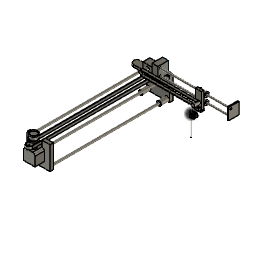
2 D PLOTTER v1 (Autodesk Fusion 360 design; units mm, degrees)
Autodesk Fusion 360 part; units mm, degrees
sketch "Sketch1" plane through (0, 0, 0) normal (0, 1, 0) x (1, 0, 0)
  line L0 (0, 0) -> (100, 0)
  line L1 (100, 0) -> (100, 100)
  line L2 (100, 100) -> (0, 100)
  line L3 (0, 100) -> (0, 0)
  dimension "d1" = 100
  dimension "d2" = 100
  constraint coincident L0.start L3.end
  constraint horizontal L0
  constraint perpendicular L0 L1
  constraint perpendicular L1 L2
  constraint perpendicular L0 L3
  measures "d1" distance of L0.start L0.end
  measures "d2" distance of L0.end L1.end
extrude "Extrude1" add sketch "Sketch1" along normal blind 15 makes body 1
sketch "Sketch2" plane through (0, 0, 0) normal (0, -1, 0) x (1, 0, 0)
  line L0 (0, 0) -> (0, -100)
  line L1 (0, -100) -> (100, -100)
  line L2 (100, -100) -> (100, 0)
  line L3 (100, 0) -> (0, 0)
  line L4 (35, -25) -> (65, -25)
  line L5 (75, -75) -> (75, -35)
  line L6 (25, -35) -> (25, -75)
  line L7 (25, -75) -> (75, -75)
  arc A0 (35, -25) -> (25, -35) centre (35, -35) ccw
  arc A1 (75, -35) -> (65, -25) centre (65, -35) ccw
  dimension "d5" = 10
  constraint parallel L1 L4
  constraint perpendicular L4 L5
  constraint perpendicular L4 L6
  constraint perpendicular L5 L7
  constraint tangent L4 A0
  constraint tangent L6 A0
  constraint tangent L4 A1
  constraint tangent L5 A1
  constraint equal A0 A1
  measures "d5" radius of A0
extrude "Extrude2" add sketch "Sketch2" along normal blind 40 contours L4 L5 L6 L7 A0 A1 bodies 1
sketch "Sketch3" plane through (0, 0, -25) normal (0, 0, 1) x (-1, 0, 0)
  line L0 (-65, 0) -> (-35, 0)
  line L1 (-35, 0) -> (-35, 40)
  line L2 (-35, 40) -> (-65, 40)
  line L3 (-65, 40) -> (-65, 0)
  circle A0 centre (-50, 20) radius 10
  dimension "d8" = 20
  measures "d8" diameter of A0
extrude "Extrude3" add sketch "Sketch3" along normal blind 30 contours A0 bodies 1
sketch "Sketch4" plane through (0, 0, 5) normal (0, 0, 1) x (-1, 0, 0)
  circle A0 centre (-50, 20) radius 10
  circle A1 centre (-50, 20) radius 15
  dimension "d11" = 30
  constraint concentric A0 A1
  measures "d11" diameter of A1
extrude "Extrude4" add sketch "Sketch4" along normal blind 20 contours A0 | A1 bodies 1
sketch "Sketch5" plane through (0, 0, 25) normal (0, 0, 1) x (-1, 0, 0)
  circle A0 centre (-50, 20) radius 15
  circle A1 centre (-50, 20) radius 16.5
  dimension "d14" = 33
  constraint concentric A0 A1
  measures "d14" diameter of A1
extrude "Extrude5" add sketch "Sketch5" along normal blind 5 separate body makes body 2
sketch "Sketch6" plane through (0, 0, 5) normal (0, 0, -1) x (1, 0, 0)
  circle A0 centre (50, 20) radius 15
  circle A1 centre (50, 20) radius 10
  circle A2 centre (50, 21.7995) radius 17.5
  dimension "d17" = 35
  measures "d17" diameter of A2
extrude "Extrude6" add sketch "Sketch6" against normal blind 5 contours A2 bodies 1
sketch "Sketch7" plane through (0, 15, 0) normal (0, 1, 0) x (-1, 0, 0)
  line L0 (0, -100) -> (0, 0)
  line L1 (0, 0) -> (-100, 0)
  line L2 (-100, 0) -> (-100, -100)
  line L3 (-100, -100) -> (0, -100)
  circle A0 centre (-90, -10) radius 5
  circle A1 centre (-10, -10) radius 5
  circle A2 centre (-90, -90) radius 5
  circle A3 centre (-10, -90) radius 5
  dimension "d20" = 10
  dimension "d21" = 10
  dimension "d22" = 10
  dimension "d23" = 10
  measures "d20" diameter of A0
  measures "d21" diameter of A1
  measures "d22" diameter of A2
  measures "d23" diameter of A3
extrude "Extrude7" add sketch "Sketch7" along normal blind 500 contours A0 | A1 | A2 | A3 bodies 1
sketch "Sketch8" plane through (0, 515, 0) normal (0, 1, 0) x (-1, 0, 0)
  circle A0 centre (-10, -10) radius 5
  line L0 (0, 0) -> (0, -97.104)
  line L1 (0, -100) -> (-100, -100)
  line L2 (-100, -100) -> (-100, 0)
  line L3 (-100, 0) -> (0, 0)
  line L4 (0, -100) -> (0, 0)
  dimension "d26" = 100
  dimension "d27" = 100
  dimension "d28" = 100
  dimension "d29" = 100
  constraint coincident L0.start L3.end
  constraint vertical L0
  constraint perpendicular L0 L1
  constraint perpendicular L1 L2
  constraint perpendicular L2 L3
  constraint perpendicular L1 L4
  measures "d26" distance of L1.start L1.end
  measures "d27" distance of L1.end L2.end
  measures "d28" distance of L2.end L0.start
  measures "d29" distance of L1.start L0.start
extrude "Extrude8" add sketch "Sketch8" along normal blind 15 separate body makes body 3
sketch "Sketch9" plane through (0, 515, 0) normal (0, 1, 0) x (-1, 0, 0)
  circle A0 centre (-10, -10) radius 5
  circle A1 centre (-10, -10) radius 10
  circle A2 centre (-10, -10) radius 6
  dimension "d32" = 20
  dimension "d33" = 12
  constraint concentric A0 A1
  constraint concentric A1 A2
  measures "d32" diameter of A1
  measures "d33" diameter of A2
extrude "Extrude9" add sketch "Sketch9" against normal blind 35 contours A1 bodies 3
sketch "Sketch10" plane through (0, 515, 0) normal (0, 1, 0) x (-1, 0, 0)
  circle A0 centre (-10, -90) radius 5
  circle A1 centre (-10, -90) radius 6
  circle A2 centre (-10, -90) radius 10
  dimension "d36" = 12
  dimension "d37" = 20
  constraint concentric A0 A1
  constraint concentric A1 A2
  measures "d36" diameter of A1
  measures "d37" diameter of A2
extrude "Extrude10" add sketch "Sketch10" against normal blind 35 contours A2 bodies 3
sketch "Sketch11" plane through (0, 515, 0) normal (0, -1, 0) x (1, 0, 0)
  arc A0 (10, -100) -> (0, -90) centre (10, -90) ccw
  line L0 (10, -100) -> (100, -100)
  line L1 (100, -100) -> (100, 0)
  line L2 (100, 0) -> (10, 0)
  arc A1 (0, -10) -> (10, 0) centre (10, -10) ccw
  line L3 (0, -10) -> (0, -90)
  circle A2 centre (90, -10) radius 6
  circle A3 centre (90, -10) radius 10
  circle A4 centre (90, -90) radius 6
  circle A5 centre (90, -90) radius 10
  dimension "d40" = 12
  dimension "d41" = 20
  dimension "d42" = 12
  dimension "d43" = 20
  constraint concentric A2 A3
  constraint concentric A4 A5
  measures "d40" diameter of A2
  measures "d41" diameter of A3
  measures "d42" diameter of A4
  measures "d43" diameter of A5
extrude "Extrude11" add sketch "Sketch11" along normal blind 35 contours A5 | A3 bodies 3
sketch "Sketch12" plane through (0, 0, 0) normal (0, 0, 1) x (-1, 0, 0)
  line L0 (-90, -515) -> (-100, -515)
  line L1 (-100, -515) -> (-100, -530)
  line L2 (-100, -530) -> (0, -530)
  line L3 (0, -530) -> (0, -515)
  line L4 (0, -515) -> (-10, -515)
  line L5 (-10, -515) -> (-90, -515)
  line L6 (-110, -470) -> (10, -470)
  arc A0 (10, -500) -> (10, -470) centre (10, -485) ccw
  line L7 (10, -500) -> (-110, -500)
  arc A1 (-110, -470) -> (-110, -500) centre (-110, -485) ccw
  constraint horizontal L6
  constraint tangent L6 A0
  constraint tangent A0 L7
  constraint parallel L6 L7
  constraint tangent L7 A1
  constraint tangent L6 A1
extrude "Extrude12" add sketch "Sketch12" along normal blind 10 separate body contours L6 A0 L7 A1 makes body 4
sketch "Sketch13" plane through (0, 0, 0) normal (0, 0, -1) x (1, 0, 0)
  arc A0 (-10, -470) -> (-10, -500) centre (-10, -485) ccw
  line L0 (-10, -500) -> (110, -500)
  arc A1 (110, -500) -> (110, -470) centre (110, -485) ccw
  line L1 (110, -470) -> (-10, -470)
  line L2 (40, -475) -> (60, -475)
  line L3 (60, -475) -> (60, -495)
  line L4 (60, -495) -> (40, -495)
  line L5 (40, -495) -> (40, -475)
  constraint parallel L0 L2
  constraint perpendicular L2 L3
  constraint perpendicular L3 L4
  constraint perpendicular L2 L5
extrude "Extrude13" add sketch "Sketch13" along normal blind 10 contours L2 L3 L4 L5 bodies 4
sketch "Sketch14" plane through (0, 530, 0) normal (0, 1, 0) x (-1, 0, 0)
  circle A0 centre (-10, -10) radius 5
  line L0 (-100, -100) -> (0, -100)
  line L1 (0, -100) -> (0, 0)
  line L2 (0, 0) -> (-100, 0)
  line L3 (-100, 0) -> (-100, -100)
  line L4 (-65, -25) -> (-65, 0)
  line L5 (-65, 0) -> (-35, 0)
  line L6 (-35, -25) -> (-35, 0)
  line L7 (-65, -25) -> (-35, -25)
  constraint coincident L2 L4.end
  constraint perpendicular L2 L4
  constraint coincident L2 L5.end
  constraint perpendicular L5 L6
  constraint perpendicular L6 L7
extrude "Extrude14" cut sketch "Sketch14" against normal blind 15 contours L2 L4 L5 L6 L7 bodies 3
sketch "Sketch15" plane through (0, 15, 0) normal (0, 1, 0) x (-1, 0, 0)
  circle A0 centre (-90, -90) radius 5
  circle A1 centre (-90, -10) radius 5
  circle A2 centre (-10, -90) radius 5
  circle A3 centre (-10, -10) radius 5
  line L0 (0, -100) -> (0, 0)
  line L1 (0, 0) -> (-100, 0)
  line L2 (-100, 0) -> (-100, -100)
  line L3 (-100, -100) -> (0, -100)
  line L4 (-65.2249, 0) -> (-65.2249, -24.1277)
  line L5 (-65.2249, 0) -> (-65.2249, -25)
  line L6 (-65.2249, -25) -> (-35, -25)
  line L7 (-35, -25) -> (-35, 0)
  line L8 (-65.2249, 0) -> (-35, 0)
  constraint coincident L1 L4.start
  constraint perpendicular L1 L4
  constraint perpendicular L1 L5
  constraint perpendicular L5 L6
  constraint coincident L1 L7.end
  constraint perpendicular L1 L7
extrude "Extrude15" cut sketch "Sketch15" against normal blind 15 contours L1 L4 L5 L6 L7 L8 bodies 1
sketch "Sketch16" plane through (0, -40, 0) normal (0, -1, 0) x (1, 0, 0)
  arc A0 (35, -25) -> (25, -35) centre (35, -35) ccw
  line L0 (25, -35) -> (25, -75)
  line L1 (25, -75) -> (75, -75)
  line L2 (75, -75) -> (75, -35)
  arc A1 (75, -35) -> (65, -25) centre (65, -35) ccw
  line L3 (65, -25) -> (35, -25)
  line L4 (37, -3) -> (39, -3)
  line L5 (39, -3) -> (39, -15)
  line L6 (39, -15) -> (37, -15)
  line L7 (37, -15) -> (37, -3)
  line L8 (61, -3) -> (63, -3)
  line L9 (63, -3) -> (63, -15)
  line L10 (63, -15) -> (61, -15)
  line L11 (61, -15) -> (61, -3)
  dimension "d54" = 2
  constraint parallel L3 L4
  constraint perpendicular L4 L5
  constraint perpendicular L5 L6
  constraint perpendicular L4 L7
  constraint horizontal L8
  constraint coincident L8 L9.start
  constraint perpendicular L8 L9
  constraint perpendicular L9 L10
  constraint perpendicular L8 L11
  measures "d54" distance of L4.start L4.end
extrude "Extrude16" add sketch "Sketch16" against normal blind 570 separate body contours L4 L5 L6 L7 | L8 L9 L10 L11 makes body 5 at (39, 150, -7) makes body 6 at (63, 150, -7)
sketch "Sketch17" plane through (0, 0, -3) normal (0, 0, 1) x (-1, 0, 0)
  line L0 (-37, 40) -> (-39, 40)
  line L1 (-39, 40) -> (-39, -530)
  line L2 (-39, -530) -> (-37, -530)
  line L3 (-37, -530) -> (-37, 40)
  circle A0 centre (-50, 40) radius 13
  line L4 (-37, 40) -> (-63, 40)
  circle A1 centre (-50, 40) radius 11
  constraint coincident L0.start L3.end
  constraint coincident A0 L4.end
  constraint perpendicular L3 L4
  constraint concentric A0 A1
extrude "Extrude17" add sketch "Sketch17" against normal blind 12 contours L0 A0 L4 A1 bodies 5 6
sketch "Sketch18" plane through (0, 0, -25) normal (0, 0, 1) x (-1, 0, 0)
  line L0 (-65, -530) -> (-35, -530)
  line L1 (-35, -530) -> (-35, -515)
  line L2 (-35, -515) -> (-65, -515)
  line L3 (-65, -515) -> (-65, -530)
  circle A0 centre (-50, -522.072) radius 10.861
extrude "Extrude18" add sketch "Sketch18" along normal blind 35 contours L0 L2 A0 | L0 A0 | L2 A0 bodies 3
sketch "Sketch19" plane through (0, 0, -3) normal (0, 0, 1) x (-1, 0, 0)
  line L0 (-39, 40) -> (-39, -530)
  line L1 (-39, -530) -> (-37, -530)
  line L2 (-37, -530) -> (-37, 40)
  arc A0 (-37, 40) -> (-63, 40) centre (-50, 40) ccw
  line L3 (-63, 40) -> (-63, -530)
  line L4 (-63, -530) -> (-61, -530)
  line L5 (-61, -530) -> (-61, 40)
  arc A1 (-39, 40) -> (-61, 40) centre (-50, 40) ccw
  circle A2 centre (-50, -530) radius 15
  circle A3 centre (-50, -530) radius 13
  line L6 (-65, -530) -> (-35, -530)
  line L7 (-35, -530) -> (-65, -530)
  constraint concentric A2 A3
  constraint tangent L2 A3
  constraint coincident A2 L6.start
  constraint perpendicular L2 L6
  constraint parallel L6 L7
extrude "Extrude19" add sketch "Sketch19" against normal blind 15 separate body contours A2 A3 L6 L7 makes body 7
sketch "Sketch20" plane through (0, 0, 0) normal (1, 0, 0) x (0, 1, 0)
sketch "Sketch21" plane through (100, 0, 0) normal (1, 0, 0) x (0, 1, 0)
  line L0 (515, -90) -> (515, -100)
  line L1 (515, -100) -> (530, -100)
  line L2 (530, -100) -> (530, 0)
  line L3 (530, 0) -> (515, 0)
  line L4 (515, 0) -> (515, -10)
  line L5 (515, -10) -> (515, -90)
  line L6 (470, 40) -> (500, 40)
  line L7 (500, 40) -> (500, 10)
  line L8 (500, 10) -> (470, 10)
  line L9 (470, 10) -> (470, 40)
  constraint horizontal L6
  constraint perpendicular L6 L7
  constraint perpendicular L7 L8
  constraint perpendicular L6 L9
extrude "Extrude20" add sketch "Sketch21" against normal blind 70 contours L6 L7 L8 L9 bodies 4
sketch "Sketch22" plane through (100, 0, 0) normal (1, 0, 0) x (0, 1, 0)
  line L0 (470, 10) -> (500, 10)
  line L1 (500, 10) -> (500, 40)
  line L2 (500, 40) -> (470, 40)
  line L3 (470, 40) -> (470, 10)
  line L4 (470, 10) -> (465, 10)
  line L5 (465, 10) -> (465, 60)
  line L6 (465, 60) -> (510, 60)
  line L7 (510, 60) -> (510, 10)
  line L8 (510, 10) -> (500, 10)
  dimension "d65" = 50
  constraint coincident L0.start L3.end
  constraint perpendicular L3 L4
  constraint perpendicular L0 L5
  constraint perpendicular L5 L6
  constraint perpendicular L0 L7
  constraint coincident L0.end L1.start
  constraint perpendicular L1 L8
  measures "d65" distance of L4.end L5.end
extrude "Extrude21" add sketch "Sketch22" against normal blind 25 contours L1 L2 L3 L4 L5 L6 L7 L8 bodies 4
sketch "Sketch23" plane through (0, 470, 0) normal (0, -1, 0) x (1, 0, 0)
  line L0 (100, 10) -> (75, 10)
  line L1 (75, 10) -> (75, 40)
  line L2 (75, 40) -> (30, 40)
  line L3 (30, 40) -> (30, 10)
  line L4 (30, 10) -> (-10, 10)
  line L5 (-10, 10) -> (-10, 0)
  line L6 (-10, 0) -> (110, 0)
  line L7 (110, 0) -> (110, 10)
  line L8 (110, 10) -> (100, 10)
  circle A0 centre (50, 25) radius 7.5
  dimension "d68" = 15
  measures "d68" diameter of A0
extrude "Extrude22" add sketch "Sketch23" along normal blind 30 contours A0 bodies 4
sketch "Sketch24" plane through (100, 0, 0) normal (1, 0, 0) x (0, 1, 0)
  line L0 (470, 10) -> (500, 10)
  line L1 (500, 10) -> (510, 10)
  line L2 (510, 10) -> (510, 60)
  line L3 (510, 60) -> (465, 60)
  line L4 (465, 60) -> (465, 10)
  line L5 (465, 10) -> (470, 10)
  circle A0 centre (475, 50) radius 4
  circle A1 centre (475, 20) radius 4
  dimension "d71" = 8
  dimension "d72" = 8
  measures "d71" diameter of A0
  measures "d72" diameter of A1
extrude "Extrude23" add sketch "Sketch24" along normal blind 200 contours A0 | A1 bodies 4
sketch "Sketch25" plane through (0, 510, 0) normal (0, 1, 0) x (-1, 0, 0)
  line L0 (-100, 60) -> (-100, 10)
  line L1 (-100, 10) -> (-75, 10)
  line L2 (-75, 10) -> (-75, 60)
  line L3 (-75, 60) -> (-100, 60)
sketch "Sketch26" plane through (300, 0, 0) normal (1, 0, 0) x (0, 1, 0)
  circle A0 centre (475, 20) radius 4
  circle A1 centre (475, 50) radius 5
  circle A2 centre (475, 20) radius 5
  circle A3 centre (475, 20) radius 10
  circle A4 centre (475, 50) radius 10
  dimension "d75" = 10
  dimension "d76" = 10
  dimension "d77" = 20
  dimension "d78" = 20
  constraint concentric A0 A2
  constraint concentric A0 A3
  constraint concentric A1 A4
  measures "d75" diameter of A1
  measures "d76" diameter of A2
  measures "d77" diameter of A3
  measures "d78" diameter of A4
extrude "Extrude24" add sketch "Sketch26" against normal blind 30 separate body contours A3 | A4 makes body 8 at (280, 484.9503, 19.0043) makes body 9 at (280, 484.9503, 49.0043)
sketch "Sketch27" plane through (300, 0, 0) normal (1, 0, 0) x (0, 1, 0)
  circle A0 centre (475, 50) radius 4
  circle A1 centre (475, 50) radius 4
  circle A2 centre (475, 20) radius 4
  dimension "d81" = 8
  dimension "d82" = 8
  constraint concentric A0 A1
  measures "d81" diameter of A1
  measures "d82" diameter of A2
extrude "Extrude25" add sketch "Sketch27" along normal blind 100 bodies 4
sketch "Sketch28" plane through (0, 465, 0) normal (0, -1, 0) x (1, 0, 0)
  line L0 (100, 10) -> (100, 60)
  line L1 (100, 60) -> (75, 60)
  line L2 (75, 60) -> (75, 10)
  line L3 (75, 10) -> (100, 10)
  line L4 (272, 70) -> (298, 70)
  line L5 (298, 70) -> (298, 0)
  line L6 (298, 0) -> (272, 0)
  line L7 (272, 0) -> (272, 70)
  constraint horizontal L4
  constraint vertical L5
  constraint horizontal L6
  constraint vertical L7
extrude "Extrude26" add sketch "Sketch28" along normal blind 10 separate body contours L4 L5 L6 L7 makes body 10
sketch "Sketch29" plane through (0, 0, 0) normal (0, 0, -1) x (1, 0, 0)
  line L0 (272, -465) -> (298, -465)
  line L1 (298, -465) -> (298, -455)
  line L2 (298, -455) -> (272, -455)
  line L3 (272, -455) -> (272, -465)
  line L4 (275, -455) -> (295, -455)
  line L5 (295, -455) -> (295, -445)
  line L6 (295, -445) -> (275, -445)
  line L7 (275, -445) -> (275, -455)
  line L8 (280, -450) -> (290.3436, -450)
  line L9 (290.3436, -450) -> (290.3436, -461.9847)
  line L10 (290.3436, -461.9847) -> (280, -461.9847)
  line L11 (280, -461.9847) -> (280, -450)
  constraint horizontal L4
  constraint vertical L5
  constraint horizontal L6
  constraint vertical L7
  constraint coincident L2 L4.start
  constraint horizontal L8
  constraint vertical L9
  constraint horizontal L10
  constraint vertical L11
extrude "Extrude27" add sketch "Sketch29" against normal blind 10 contours L2 L4 L5 L6 L7 L8 L9 L11 bodies 10
sketch "Sketch30" plane through (0, 0, 0) normal (0, 0, -1) x (1, 0, 0)
  line L0 (290.3436, -455) -> (280, -455)
  line L1 (280, -455) -> (280, -450)
  line L2 (280, -450) -> (290.3436, -450)
  line L3 (290.3436, -450) -> (290.3436, -455)
  line L4 (295, -455) -> (295, -445)
  line L5 (295, -445) -> (275, -445)
  line L6 (275, -445) -> (275, -455)
  line L7 (275, -455) -> (272, -455)
  line L8 (272, -455) -> (272, -465)
  line L9 (272, -465) -> (298, -465)
  line L10 (298, -465) -> (298, -455)
  line L11 (298, -455) -> (295, -455)
  line L12 (277.6152, -455) -> (293.6015, -455)
  line L13 (293.6015, -455) -> (293.6015, -470.4905)
  line L14 (293.6015, -470.4905) -> (277.6152, -470.4905)
  line L15 (277.6152, -470.4905) -> (277.6152, -455)
  constraint horizontal L12
  constraint vertical L13
  constraint horizontal L14
  constraint vertical L15
extrude "Extrude28" add sketch "Sketch30" along normal blind 10 contours L0 L9 L12 L13 L15 | L9 L13 L14 L15 bodies 10
sketch "Sketch31" plane through (0, 455, 0) normal (0, -1, 0) x (1, 0, 0)
  line L0 (295, 10) -> (295, 0)
  line L1 (295, 0) -> (298, 0)
  line L2 (298, 0) -> (298, 70)
  line L3 (298, 70) -> (272, 70)
  line L4 (272, 70) -> (272, 0)
  line L5 (272, 0) -> (275, 0)
  line L6 (275, 0) -> (275, 10)
  line L7 (275, 10) -> (280, 10)
  line L8 (280, 10) -> (280, 0)
  line L9 (280, 0) -> (277.6152, 0)
  line L10 (277.6152, 0) -> (277.6152, -10)
  line L11 (277.6152, -10) -> (293.6015, -10)
  line L12 (293.6015, -10) -> (293.6015, 0)
  line L13 (293.6015, 0) -> (290.3436, 0)
  line L14 (290.3436, 0) -> (290.3436, 10)
  line L15 (290.3436, 10) -> (295, 10)
  circle A0 centre (285, -5) radius 3
  dimension "d91" = 6
  measures "d91" diameter of A0
extrude "Extrude29" add sketch "Sketch31" along normal blind 25 contours A0 bodies 10
sketch "Sketch32" plane through (0, 430, 0) normal (0, -1, 0) x (1, 0, 0)
  circle A0 centre (285, -5) radius 3
  circle A1 centre (297, -5) radius 9
  constraint tangent A0 A1
extrude "Extrude30" add sketch "Sketch32" against normal blind 2 separate body contours A1 makes body 11
sketch "Sketch33" plane through (0, 430, 0) normal (0, -1, 0) x (1, 0, 0)
  circle A0 centre (297, -5) radius 9
  line L0 (278.2063, 5.2233) -> (295, 5.2233)
  line L1 (295, 5.2233) -> (295, -20)
  line L2 (295, -20) -> (278.2063, -20)
  line L3 (278.2063, -20) -> (278.2063, 5.2233)
  constraint horizontal L0
  constraint vertical L1
  constraint horizontal L2
  constraint vertical L3
extrude "Extrude31" add sketch "Sketch33" along normal blind 5 contours A0 L1 | A0 L0 L1 L2 L3 picked at (293.4679, -7.0409) bodies 10 11
sketch "Sketch34" plane through (0, 425, 0) normal (0, -1, 0) x (1, 0, 0)
  line L0 (278.2063, -20) -> (295, -20)
  line L1 (295, -20) -> (295, 5.2233)
  line L2 (295, 5.2233) -> (278.2063, 5.2233)
  line L3 (278.2063, 5.2233) -> (278.2063, -20)
  line L4 (282, -2) -> (291, -2)
  line L5 (291, -2) -> (291, -15)
  line L6 (291, -15) -> (282, -15)
  line L7 (282, -15) -> (282, -2)
  constraint horizontal L4
  constraint vertical L5
  constraint horizontal L6
  constraint vertical L7
extrude "Extrude32" add sketch "Sketch34" along normal blind 6 separate body contours L4 L5 L6 L7 makes body 12
sketch "Sketch35" plane through (0, 0, -2) normal (0, 0, 1) x (-1, 0, 0)
  line L0 (-291, -425) -> (-282, -425)
  line L1 (-282, -425) -> (-282, -419)
  line L2 (-282, -419) -> (-291, -419)
  line L3 (-291, -419) -> (-291, -425)
  circle A0 centre (-286.1909, -421.937) radius 1.5
  dimension "d101" = 3
  measures "d101" diameter of A0
extrude "Extrude33" cut sketch "Sketch35" against normal blind 21 contours A0 bodies 12
sketch "Sketch36" plane through (0, 0, -2) normal (0, 0, 1) x (-1, 0, 0)
  circle A0 centre (-286.1909, -421.937) radius 1.5
  line L0 (-291, -425) -> (-282, -425)
  line L1 (-282, -425) -> (-282, -419)
  line L2 (-282, -419) -> (-291, -419)
  line L3 (-291, -419) -> (-291, -425)
  circle A1 centre (-286.1909, -421.937) radius 1.25
  dimension "d104" = 2.5
  constraint concentric A0 A1
  measures "d104" diameter of A1
sketch "Sketch37" plane through (0, 0, -15) normal (0, 0, -1) x (1, 0, 0)
  circle A0 centre (286.1909, -421.937) radius 1.5
  line L0 (282, -425) -> (291, -425)
  line L1 (291, -425) -> (291, -419)
  line L2 (291, -419) -> (282, -419)
  line L3 (282, -419) -> (282, -425)
  circle A1 centre (286.1909, -421.937) radius 1.25
  dimension "d105" = 2.5
  constraint concentric A0 A1
  measures "d105" diameter of A1
extrude "Extrude34" add sketch "Sketch37" along normal blind 75 and the other way blind 50 separate body contours A1 makes body 13
sketch "Sketch38" plane through (0, 0, -90) normal (0, 0, -1) x (1, 0, 0)
  circle A0 centre (286.1909, -421.937) radius 1.25
  circle A1 centre (286.1909, -421.937) radius 1.25
  dimension "d110" = 2.5
  constraint concentric A0 A1
  measures "d110" diameter of A1
extrude "Extrude35" add sketch "Sketch38" along normal blind 4 draft -15 bodies 13
sketch "Sketch39" plane through (0, 440, 0) normal (0, -1, 0) x (1, 0, 0)
  circle A0 centre (50, 25) radius 7.5
  circle A1 centre (286, 25) radius 7.5
  dimension "d113" = 15
  measures "d113" diameter of A1
extrude "Extrude36" add sketch "Sketch39" along normal blind 10 and the other way blind 15 separate body contours A1 makes body 14
sketch "Sketch40" plane through (0, 0, 0) normal (0, 1, 0) x (1, 0, 0)
sketch "Sketch41" plane through (30, 0, 0) normal (-1, 0, 0) x (0, -1, 0)
  line L0 (-500, 10) -> (-470, 10)
  line L1 (-470, 10) -> (-470, 40)
  line L2 (-470, 40) -> (-500, 40)
  line L3 (-500, 40) -> (-500, 10)
  line L4 (-450, 36) -> (-439, 36)
  line L5 (-439, 36) -> (-439, 34)
  line L6 (-439, 34) -> (-450, 34)
  line L7 (-450, 34) -> (-450, 36)
  line L8 (-450, 16) -> (-439, 16)
  line L9 (-439, 16) -> (-439, 14)
  line L10 (-439, 14) -> (-450, 14)
  line L11 (-450, 14) -> (-450, 16)
  constraint horizontal L4
  constraint vertical L5
  constraint horizontal L6
  constraint vertical L7
  constraint horizontal L8
  constraint vertical L9
  constraint horizontal L10
  constraint vertical L11
extrude "Extrude37" add sketch "Sketch41" along normal blind -260 and the other way blind 20 separate body contours L4 L5 L6 L7 | L8 L9 L10 L11 makes body 15 at (130, 446.3333, 36) makes body 16 at (130, 446.3333, 16)
sketch "Sketch42" plane through (400, 0, 0) normal (1, 0, 0) x (0, 1, 0)
  circle A0 centre (475, 50) radius 4
  line L0 (465, 60) -> (510, 60)
  line L1 (510, 60) -> (510, 10)
  line L2 (510, 10) -> (465, 10)
  line L3 (465, 10) -> (465, 60)
  constraint horizontal L0
  constraint vertical L1
  constraint horizontal L2
  constraint vertical L3
extrude "Extrude38" add sketch "Sketch42" along normal blind 5 separate body makes body 17
